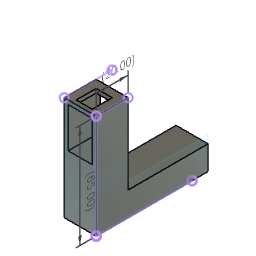
mitad proyecto v3 (Autodesk Fusion 360 design; units mm, degrees)
Autodesk Fusion 360 part; units mm, degrees
sketch "Boceto1" plane through (0, 0, 0) normal (0, 0, 1) x (1, 0, 0)
  line L0 (0, 0) -> (20, 0)
  line L1 (20, 0) -> (20, 30)
  line L2 (20, 30) -> (0, 30)
  line L3 (0, 30) -> (0, 0)
  dimension "d1" = 20
  dimension "d2" = 30
  constraint horizontal L0
  constraint vertical L1
  constraint horizontal L2
  constraint vertical L3
  constraint coincident L0.start L3.end
  measures "d1" distance of L1.end L2.end
  measures "d2" distance of L0.end L1.end
extrude "Extruir1" add sketch "Boceto1" along normal blind 20
extrude "Extruir2" add 1 faces at (13.3333, 30, 6.6667) along direction (0, 1, 0) blind 20
sketch "Boceto2" plane through (0, 0, 0) normal (0, 0, 1) x (1, 0, 0)
  line L0 (20, 0, 20) -> (0, 0, 20)
  line L1 (0, 0, 20) -> (0, 30, 20)
  line L2 (0, 30, 20) -> (20, 30, 20)
  line L3 (20, 30, 20) -> (20, 0, 20)
  dimension "d7" = 30
  dimension "d8" = 20
extrude "Extruir3" add sketch "Boceto2" along normal blind 45 contours L0 L1 L2 L3 in plane through (0, 0, 20) normal (0, 0, 1)
extrude "Extruir4" add 1 faces at (13.3333, 50, 6.6667) along direction (0, 1, 0) blind 10
sketch "Boceto3" plane through (0, 0, 0) normal (0, 0, 1) x (1, 0, 0)
  line L0 (20, 0) -> (20, 60)
  dimension "d13" = 60
  measures "d13" distance of L0.start L0.end
extrude "Extruir5" add 1 faces at (13.3333, 60, 6.6667) along direction (0, 1, 0) blind 10
sketch "Boceto4" plane through (0, 0, 0) normal (0, 0, 1) x (1, 0, 0)
sketch "Boceto5" plane through (0, 0, 0) normal (1, 0, 0) x (0, 1, 0)
  line L0 (0, 65) -> (30, 65)
  dimension "d16" = 30
  measures "d16" distance of L0.start L0.end
extrude "Extruir6" cut 1 faces at (6.6667, 30, 35) along direction (0, -1, 0) blind 10
sketch "Boceto6" plane through (0, 0, 0) normal (0, 1, 0) x (1, 0, 0)
  line L0 (17.5, -62.5) -> (2.5, -62.5)
  line L1 (2.5, -62.5) -> (2.5, -39.5)
  line L2 (2.5, -39.5) -> (17.5, -39.5)
  line L3 (17.5, -39.5) -> (17.5, -62.5)
  dimension "d19" = 15
  dimension "d20" = 23
  constraint horizontal L0
  constraint vertical L1
  constraint horizontal L2
  constraint vertical L3
  measures "d19" distance of L0.start L0.end
  measures "d20" distance of L0.end L1.end
extrude "Extruir7" cut sketch "Boceto6" along normal blind 33
hole "Agujero1" at (9.9694, 20, 63.7746) direction (0, -1, 0) diameter 1 depth 4 tip angle 118
hole "Agujero2" at (10.0421, 20, 38.3) direction (0, -1, 0) diameter 1 depth 4 tip angle 118
sketch "Boceto7" plane through (0, 0, 20) normal (0, 0, 1) x (-1, 0, 0)
  line L0 (-20, -20) -> (-20, -70)
  line L1 (-20, -70) -> (0, -70)
  line L2 (0, -70) -> (0, -20)
  line L3 (0, -20) -> (-20, -20)
sketch "Boceto8" plane through (0, 0, 0) normal (0, 0, 1) x (1, 0, 0)
  line L0 (13.5, 70) -> (6.5, 70)
  line L1 (6.5, 70) -> (6.5, 40)
  line L2 (6.5, 40) -> (13.5, 40)
  line L3 (13.5, 40) -> (13.5, 70)
  dimension "d29" = 30
  dimension "d30" = 7
  constraint horizontal L0
  constraint vertical L1
  constraint horizontal L2
  constraint vertical L3
  measures "d29" distance of L0.start L2.end
  measures "d30" distance of L0.start L0.end
extrude "Extruir8" cut sketch "Boceto8" along normal blind 3
sketch "Boceto9" plane through (0, 0, 0) normal (0, 0, -1) x (1, 0, 0)
  line L0 (13.5, -40) -> (13.5, -70)
  line L1 (13.5, -70) -> (20, -70)
  line L2 (20, -70) -> (20, 0)
  line L3 (20, 0) -> (0, 0)
  line L4 (0, 0) -> (0, -70)
  line L5 (0, -70) -> (6.5, -70)
  line L6 (6.5, -70) -> (6.5, -40)
  line L7 (6.5, -40) -> (13.5, -40)
  line L8 (13.5, -70) -> (12, -70)
  line L9 (12, -70) -> (12, -40)
  line L10 (12, -40) -> (13.5, -40)
  line L11 (13.5, -40) -> (13.5, -70)
  line L12 (6.5, -40) -> (8, -40)
  line L13 (8, -40) -> (8, -70)
  line L14 (8, -70) -> (6.5, -70)
  line L15 (6.5, -70) -> (6.5, -40)
  constraint horizontal L8
  constraint vertical L9
  constraint horizontal L10
  constraint vertical L11
  constraint coincident L7 L9.end
  constraint coincident L0.end L1.start
  constraint horizontal L12
  constraint vertical L13
  constraint horizontal L14
  constraint vertical L15
  constraint coincident L6.end L7.start
extrude "Extruir9" add sketch "Boceto9" against normal blind 1 contours L0 L7 L8 L9 L10 L11
extrude "Extruir10" add 1 faces at (8.8333, 60, 3) along direction (0, 0, -1) blind 1
extrude "Extruir11" cut 1 faces at (8.8333, 60, 2) along direction (0, 0, 1) blind 2
sketch "Boceto10" plane through (0, 0, 0) normal (0, 0, -1) x (1, 0, 0)
  line L0 (12, -70) -> (20, -70)
  line L1 (20, -70) -> (20, 0)
  line L2 (20, 0) -> (0, 0)
  line L3 (0, 0) -> (0, -70)
  line L4 (0, -70) -> (6.5, -70)
  line L5 (6.5, -70) -> (6.5, -40)
  line L6 (6.5, -40) -> (12, -40)
  line L7 (12, -40) -> (12, -70)
  line L8 (6.5, -70) -> (8.1564, -70)
  line L9 (8.1564, -70) -> (8.1564, -40)
  line L10 (8.1564, -40) -> (6.5, -40)
  line L11 (6.5, -40) -> (6.5, -70)
  constraint horizontal L8
  constraint vertical L9
  constraint horizontal L10
  constraint vertical L11
  constraint coincident L6 L9.end
  constraint coincident L4.end L5.start
extrude "Extruir12" add sketch "Boceto10" against normal blind 1 contours L5 L6 L8 L9 L10 L11
sketch "Boceto11" plane through (0, 0, 65) normal (0, 0, 1) x (-1, 0, 0)
  line L0 (-20, -20) -> (0, -20)
  line L1 (0, -20) -> (0, 0)
  line L2 (0, 0) -> (-20, 0)
  line L3 (-20, 0) -> (-20, -20)
  line L4 (-15, -5) -> (-5, -5)
  line L5 (-5, -5) -> (-5, -15)
  line L6 (-5, -15) -> (-15, -15)
  line L7 (-15, -15) -> (-15, -5)
  constraint horizontal L4
  constraint vertical L5
  constraint horizontal L6
  constraint vertical L7
extrude "Extruir13" cut sketch "Boceto11" against normal blind 2 contours L4 L5 L6 L7
extrude "Extruir14" cut 1 faces at (11.6667, 8.3333, 63) along direction (0, 0, -1) blind 1
sketch "Boceto12" plane through (20, 0, 0) normal (1, 0, 0) x (0, 1, 0)
  line L0 (20, 20) -> (20, 65)
  line L1 (20, 65) -> (0, 65)
  line L2 (0, 65) -> (0, 0)
  line L3 (0, 0) -> (70, 0)
  line L4 (70, 0) -> (70, 20)
  line L5 (70, 20) -> (20, 20)
  line L6 (0, 0) -> (60, 0)
  dimension "d45" = 65
  dimension "d47" = 20
  dimension "d48" = 45
  dimension "d49" = 20
  dimension "d50" = 60
  measures "d45" distance of L1.end L2.end
  measures "d47" distance of L0.end L1.end
  measures "d48" distance of L0.start L0.end
  measures "d49" distance of L3.end L4.end
  measures "d50" distance of L2.end L6.end
extrude "Extruir15" cut 1 faces at (11.6667, 5, 63.3333) along direction (0, -1, 0) blind 2
extrude "Extruir16" cut 1 faces at (11.6667, 3, 63.3333) along direction (0, -1, 0) blind 0.5
extrude "Extruir17" add 1 faces at (8.3333, 15, 63.3333) along direction (0, -1, 0) blind 1
extrude "Extruir18" cut 1 faces at (7.5, 6.6667, 39.5) along direction (0, 0, -1) blind 2
hole "Agujero3" at (9.9385, 20, 35.2476) direction (0, -1, 0) diameter 1.2 depth 5 tip angle 118
sketch "Boceto13" plane through (0, 0, 65) normal (0, 0, 1) x (-1, 0, 0)
  line L0 (-5, -2.5) -> (-5, -14)
  line L1 (-5, -14) -> (-15, -14)
  line L2 (-15, -14) -> (-15, -2.5)
  line L3 (-15, -2.5) -> (-5, -2.5)
  line L4 (-20, -20) -> (0, -20)
  line L5 (0, -20) -> (0, 0)
  line L6 (0, 0) -> (-20, 0)
  line L7 (-20, 0) -> (-20, -20)
sketch "Boceto14" plane through (0, 0, 0) normal (0, -1, 0) x (1, 0, 0)
  line L0 (0, 0) -> (20, 0)
  line L1 (20, 0) -> (20, 65)
  line L2 (20, 65) -> (0, 65)
  line L3 (0, 65) -> (0, 0)
  line L4 (17.5, 62.5) -> (17.5, 37.5)
  line L5 (17.5, 37.5) -> (2.5, 37.5)
  line L6 (2.5, 37.5) -> (2.5, 62.5)
  line L7 (2.5, 62.5) -> (17.5, 62.5)
sketch "Boceto15" plane through (0, 14, 0) normal (0, -1, 0) x (1, 0, 0)
  line L0 (15, 65) -> (5, 65)
  line L1 (5, 65) -> (5, 62.5)
  line L2 (5, 62.5) -> (15, 62.5)
  line L3 (15, 62.5) -> (15, 65)
sketch "Boceto16" plane through (0, 0, 65) normal (0, 0, 1) x (-1, 0, 0)
  line L0 (-15, -14) -> (-5, -14)
  line L1 (-5, -14) -> (-5, -2.5)
  line L2 (-5, -2.5) -> (-15, -2.5)
  line L3 (-15, -2.5) -> (-15, -14)
  constraint horizontal L0
  constraint vertical L1
  constraint horizontal L2
  constraint vertical L3
extrude "Extruir19" add sketch "Boceto16" against normal blind 1
extrude "Extruir20" cut sketch "Boceto13" against normal blind 3 contours L0 L1 L2 L3
extrude "Extruir21" cut sketch "Boceto15" against normal blind 1
move_face "CarasDesfase1" offset 4 1 faces at (11.6667, 2.5, 63.3333)
sketch "Boceto17" plane through (20, 0, 0) normal (1, 0, 0) x (0, 1, 0)
  line L0 (0, 65) -> (0, 0)
  line L1 (20, 65) -> (0, 65)
  dimension "d69" = 65
  dimension "d70" = 20
  measures "d69" distance of L0.start L0.end
  measures "d70" distance of L1.start L0.start
sketch "Boceto18" plane through (20, 0, 0) normal (1, 0, 0) x (0, 1, 0)
move_face "CarasDesfase2" offset -4 1 faces at (11.6667, 6.5, 63.3333)
extrude "Extruir22" cut sketch "Boceto7" against normal blind 5
sketch "Boceto19" plane through (20, 0, 0) normal (1, 0, 0) x (0, 1, 0)
sketch "Boceto20" plane through (0, 0, 0) normal (-1, 0, 0) x (0, -1, 0)
  line L0 (-20, 65) -> (-20, 15)
  line L1 (-20, 15) -> (-70, 15)
  line L2 (-70, 15) -> (-70, 0)
  line L3 (-70, 0) -> (0, 0)
  line L4 (0, 0) -> (0, 65)
  line L5 (0, 65) -> (-20, 65)
  dimension "d75" = 15
  measures "d75" distance of L1.end L2.end
sketch "Boceto21" plane through (0, 0, 0) normal (0, 0, -1) x (1, 0, 0)
  line L0 (12, -70) -> (20, -70)
  line L1 (20, -70) -> (20, 0)
  line L2 (20, 0) -> (0, 0)
  line L3 (0, 0) -> (0, -70)
  line L4 (0, -70) -> (8.1564, -70)
  line L5 (8.1564, -70) -> (8.1564, -40)
  line L6 (8.1564, -40) -> (12, -40)
  line L7 (12, -40) -> (12, -70)
  line L8 (8.1564, -55) -> (6.5082, -55)
  line L9 (6.5082, -55) -> (6.5082, -70)
  line L10 (6.5082, -70) -> (8.1564, -70)
  line L11 (8.1564, -70) -> (8.1564, -55)
  line L12 (12, -55) -> (13.5, -55)
  line L13 (13.5, -55) -> (13.5, -70)
  line L14 (13.5, -70) -> (12, -70)
  line L15 (12, -70) -> (12, -55)
  dimension "d76" = 30
  constraint horizontal L8
  constraint vertical L9
  constraint horizontal L10
  constraint vertical L11
  constraint coincident L4 L9.end
  constraint midpoint L5 L8.start
  constraint horizontal L12
  constraint vertical L13
  constraint horizontal L14
  constraint vertical L15
  constraint coincident L0 L13.end
  constraint midpoint L7 L12.start
  measures "d76" distance of L4.end L5.end
extrude "Extruir23" cut sketch "Boceto21" against normal blind 1 contours L0 L7 L12 L13 L14 L15
sketch "Boceto22" plane through (0, 0, 0) normal (0, 0, -1) x (1, 0, 0)
  line L0 (13.5, -55) -> (13.5, -70)
  line L1 (13.5, -70) -> (20, -70)
  line L2 (20, -70) -> (20, 0)
  line L3 (20, 0) -> (0, 0)
  line L4 (0, 0) -> (0, -70)
  line L5 (0, -70) -> (8.1564, -70)
  line L6 (8.1564, -70) -> (8.1564, -40)
  line L7 (8.1564, -40) -> (12, -40)
  line L8 (12, -40) -> (12, -55)
  line L9 (12, -55) -> (13.5, -55)
  line L10 (8.1564, -55) -> (6.5021, -55)
  line L11 (6.5021, -55) -> (6.5021, -70)
  line L12 (6.5021, -70) -> (8.1564, -70)
  line L13 (8.1564, -70) -> (8.1564, -55)
  constraint horizontal L10
  constraint vertical L11
  constraint horizontal L12
  constraint vertical L13
  constraint coincident L5 L11.end
  constraint midpoint L6 L10.start
extrude "Extruir24" cut sketch "Boceto22" against normal blind 1 contours L5 L6 L10 L11 L12 L13
sketch "Boceto23" plane through (0, 70, 0) normal (0, 1, 0) x (-1, 0, 0)
  line L0 (-6.5021, 1) -> (-6.5021, 0)
  line L1 (-6.5021, 0) -> (0, 0)
  line L2 (0, 0) -> (0, 15)
  line L3 (0, 15) -> (-20, 15)
  line L4 (-20, 15) -> (-20, 0)
  line L5 (-20, 0) -> (-13.5, 0)
  line L6 (-13.5, 0) -> (-13.5, 4)
  line L7 (-13.5, 4) -> (-6.5, 4)
  line L8 (-6.5, 4) -> (-6.5, 1)
  line L9 (-6.5, 1) -> (-6.5021, 1)
  dimension "d81" = 3
  dimension "d82" = 7
  measures "d81" distance of L7.end L8.end
  measures "d82" distance of L6.end L7.end
sketch "Boceto24" plane through (0, 0, 0) normal (0, 0, 1) x (1, 0, 0)
